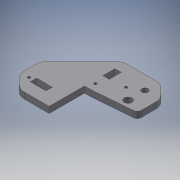
# Autodesk Inventor part: A8-0004
Saved by Autodesk Inventor 2016 SP2 (Build 200236200, 236)
## iProperties
Created: 2017-04-22
Part Number: A8-0004
Material: Generic
Document SubType Name: Modeling
Designer: EV
Density: 1 g/cm^3
Appearance: Default
Author: EV
Autodesk Inventor part; units mm, degrees
ref_plane "YZ Plane" through (0, 0, 0) normal (1, 0, 0) x (0, 1, 0)
sketch "Sketch1" plane through (0, 0, 0) normal (0, 1, 0) x (-1, 0, 0)
  line L0 (38, 0) -> (0, 0)
  line L1 (0, 0) -> (0, -45)
  line L2 (0, -45) -> (-8, -45)
  line L3 (-8, -45) -> (-63, -49.5)
  line L4 (-63, -49.5) -> (-63, -79)
  line L5 (-63, -79) -> (-46, -96)
  line L6 (-46, -96) -> (3, -96)
  line L7 (3, -96) -> (55, -44)
  line L8 (55, -44) -> (55, -17)
  line L9 (55, -17) -> (38, 0)
  line L10 (19, -15) -> (39.2, -15)
  line L11 (39.2, -15) -> (39.2, -23.2)
  line L12 (39.2, -23.2) -> (19, -23.2)
  line L13 (19, -23.2) -> (19, -15)
  line L14 (-0.3, -68) -> (-8.5, -68)
  line L15 (-8.5, -68) -> (-8.5, -83.5)
  line L16 (-8.5, -83.5) -> (-0.3, -83.5)
  line L17 (-0.3, -83.5) -> (-0.3, -68)
  dimension "d0" = 45
  dimension "d1" = 55
  dimension "d2" = 63
  dimension "d3" = 96
  dimension "d4" = 8
  dimension "d6" = 45
  dimension "d7" = 45
  dimension "d8" = 45
  dimension "d9" = 46.5
  dimension "d10" = 17
  dimension "d11" = 44
  dimension "d12" = 17
  dimension "d13" = 8.2
  dimension "d14" = 20.2
  dimension "d15" = 8.2
  dimension "d16" = 15.5
  dimension "d17" = 12.5
  dimension "d18" = 19
  dimension "d19" = 15
  dimension "d20" = 54.5
  constraints: 36 end point, 7 parallel, 4 perpendicular, 3 horizontal, 1 coincident
  measures "d0" distance of L0.end L1.end
  measures "d1" distance between parallel lines of L8 L1
  measures "d2" distance between parallel lines of L4 L1
  measures "d3" distance between parallel lines of L0 L6
  measures "d4" distance of L1.end L2.end
  measures "d6" angle of L8 L7
  measures "d7" angle of L9 L0
  measures "d8" angle of L4 L5
  measures "d9" distance from line of L3.end L6
  measures "d10" horizontal distance of L4.end L5.end
  measures "d11" distance from line of L7.end L0
  measures "d12" horizontal distance of L8.end L0.start
  measures "d13" distance between parallel lines of L12 L10
  measures "d14" distance of L11.end L12.end
  measures "d15" distance of L14.start L14.end
  measures "d16" distance of L16.end L14.start
  measures "d17" distance between parallel lines of L6 L16
  measures "d18" distance between parallel lines of L1 L13
  measures "d19" distance between parallel lines of L0 L10
  measures "d20" distance between parallel lines of L4 L15
extrude "Extrusion1" add sketch "Sketch1" along normal blind 8
fillet "Fillet1" radius 15 6 edges at (-38, 4, 0) (-55, 4, -17) (-55, 4, -44) (-3, 4, -96) (46, 4, -96) (63, 4, -79)
fillet "Fillet2" radius 5 1 edges at (63, 4, -49.5)
sketch "Sketch2" plane through (0, 8, 0) normal (0, 1, 0) x (1, 0, 0)
  arc A0 (58.4077, 49.1243) -> (63, 54.1076) centre (58, 54.1076) ccw construction
  line L0 (63, 54.1076) -> (63, 72.7868) construction
  arc A1 (63, 72.7868) -> (58.6066, 83.3934) centre (48, 72.7868) ccw construction
  line L1 (58.6066, 83.3934) -> (50.3934, 91.6066) construction
  arc A2 (50.3934, 91.6066) -> (39.7868, 96) centre (39.7868, 81) ccw construction
  line L2 (39.7868, 96) -> (3.2132, 96) construction
  arc A3 (3.2132, 96) -> (-7.3934, 91.6066) centre (3.2132, 81) ccw construction
  line L3 (-7.3934, 91.6066) -> (-50.6066, 48.3934) construction
  arc A4 (-50.6066, 48.3934) -> (-55, 37.7868) centre (-40, 37.7868) ccw construction
  line L4 (-55, 37.7868) -> (-55, 23.2132) construction
  arc A5 (-55, 23.2132) -> (-50.6066, 12.6066) centre (-40, 23.2132) ccw construction
  line L5 (-50.6066, 12.6066) -> (-42.3934, 4.3934) construction
  arc A6 (-42.3934, 4.3934) -> (-31.7868, 0) centre (-31.7868, 15) ccw construction
  line L6 (-31.7868, 0) -> (0, 0) construction
  line L7 (0, 0) -> (0, 45) construction
  line L8 (0, 45) -> (8, 45) construction
  line L9 (8, 45) -> (58.4077, 49.1243) construction
  line L10 (0.3, 68) -> (0.3, 83.5) construction
  line L11 (0.3, 83.5) -> (8.5, 83.5) construction
  line L12 (8.5, 83.5) -> (8.5, 68) construction
  line L13 (8.5, 68) -> (0.3, 68) construction
  line L14 (-39.2, 15) -> (-39.2, 23.2) construction
  line L15 (-39.2, 23.2) -> (-19, 23.2) construction
  line L16 (-19, 23.2) -> (-19, 15) construction
  line L17 (-19, 15) -> (-39.2, 15) construction
  line L18 (-39.2, 23.2) -> (-39.2, 15) construction
  line L19 (-39.2, 19.1) -> (-44.7, 19.1) construction
  line L20 (4.4, 54.5) -> (4.4, 68) construction
  line L21 (0.3, 68) -> (8.5, 68) construction
  line L22 (43.5, 78.5) -> (43.5, 57) construction
  line L23 (-39.2, 15) -> (-39.2, 23.2) construction
  line L24 (8.5, 68) -> (0.3, 68) construction
  point P0 (28, 70)
  dimension "d25" = 5.5
  dimension "d26" = 13.5
  dimension "d27" = 26
  dimension "d28" = 35
  dimension "d29" = 19.5
  dimension "d30" = 17.5
  dimension "d31" = 39
  constraints: 6 end point, 2 midpoint, 2 perpendicular, 1 vertical
  measures "d25" distance of L19.start L19.end
  measures "d26" distance of L20.start L20.end
  measures "d27" distance from line of L2 point (28, 70)
  measures "d28" distance from line of L0 point (28, 70)
  measures "d29" distance between parallel lines of L0 L22
  measures "d30" distance from line of L2 L22.start
  measures "d31" distance from line of L2 L22.end
hole "Hole1" at (28, 8, -70) at (4.4, 8, -54.5) at (-44.7, 8, -19.1) direction (0, -1, 0) diameter 3.5 end through all
hole "Hole2" at (43.5, 8, -78.5) direction (0, -1, 0) diameter 8 end through all
hole "Hole3" at (43.5, 8, -57) direction (0, -1, 0) diameter 10 end through all
ref_plane "Work Plane1" through (4.4, 8, -54.5) normal (1, 0, 0) x (0, 0, -1)
ref_plane "Work Plane2" through (-39.2, 8, -19.1) normal (0, 0, -1) x (-1, 0, 0)
body "Solid1"
